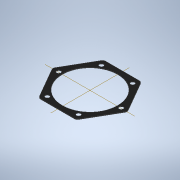
# Autodesk Inventor part: crankcase gasket
Saved by Autodesk Inventor 2021.1 (Build 251245000, 245)
## iProperties
Created: 2020-08-30
Part Number: crankcase gasket
Material: Rubber
Document SubType Name: Sheet Metal
Designer: Vamshi
Mass: 47.7006 g
Surface Area: 454.102 cm^2
Volume: 51.291 cm^3
Density: 0.93 g/cm^3
Sheet Metal Rule: Default
Appearance: Rubber - Black
Author: Vamshi
Autodesk Inventor part; units mm, degrees
ref_plane "YZ Plane" through (0, 0, 0) normal (1, 0, 0) x (0, 1, 0)
ref_plane "XZ Plane" through (0, 0, 0) normal (0, 1, 0) x (-1, 0, 0)
ref_plane "XY Plane" through (0, 0, 0) normal (0, 0, 1) x (1, 0, 0)
sketch "Sketch1" plane through (0, 0, 0) normal (0, 0, 1) x (1, 0, 0)
  line L0 (151.7796, -6.35) -> (81.3891, -128.27)
  line L1 (70.3905, -134.62) -> (-70.3905, -134.62)
  line L2 (-81.3891, -128.27) -> (-151.7796, -6.35)
  line L3 (-151.7796, 6.35) -> (-81.3891, 128.27)
  line L4 (-70.3905, 134.62) -> (70.3905, 134.62)
  line L5 (81.3891, 128.27) -> (151.7796, 6.35)
  arc A0 (-70.3905, 134.62) -> (-81.3891, 128.27) centre (-70.3905, 121.92) ccw
  arc A1 (81.3891, 128.27) -> (70.3905, 134.62) centre (70.3905, 121.92) ccw
  arc A2 (151.7796, -6.35) -> (151.7796, 6.35) centre (140.7811, 0) ccw
  arc A3 (70.3905, -134.62) -> (81.3891, -128.27) centre (70.3905, -121.92) ccw
  arc A4 (-81.3891, -128.27) -> (-70.3905, -134.62) centre (-70.3905, -121.92) ccw
  arc A5 (-151.7796, 6.35) -> (-151.7796, -6.35) centre (-140.7811, 0) ccw
  circle A6 centre (0, 0) radius 129.54 construction
  circle A7 centre (0, 0) radius 114.3
  circle A8 centre (-129.54, 0) radius 8.89
  circle A9 centre (-64.77, -112.1849) radius 8.89
  circle A10 centre (64.77, -112.1849) radius 8.89
  circle A11 centre (129.54, 0) radius 8.89
  circle A12 centre (64.77, 112.1849) radius 8.89
  circle A13 centre (-64.77, 112.1849) radius 8.89
  point P0 (155.4458, 0)
  point P1 (77.7229, -134.62)
  point P2 (-77.7229, -134.62)
  point P3 (-155.4458, 0)
  point P4 (-77.7229, 134.62)
  point P5 (77.7229, 134.62)
  dimension "d2" = 259.08
  dimension "d0" = 269.24
  dimension "d1" = 12.7
  dimension "d3" = 228.6
  dimension "d4" = 17.78
  dimension "d7" = 360
  constraints: 13 centre point, 12 end point, 12 point on circle, 12 point on line, 12 tangent, 5 equal radius, 3 coincident, 1 horizontal, 1 horizontal alignment, 28 other
  measures "d0" distance between parallel lines of L1 L4
  measures "d1" radius of A0
  measures "d3" diameter of A7
  measures "d4" diameter of A8
extrude "Extrusion1" add sketch "Sketch1" along normal blind 2.54
equation "\"BendRadius\" = Thickness"
equation "\"BendReliefWidth\" = Thickness"
equation "\"BendReliefDepth\" = 0.5 * Thickness"
equation "\"CornerReliefSize\" = 4 * Thickness"
equation "\"MinimumRemnant\" = 2 * Thickness"
equation "\"TransitionRadius\" = BendRadius"
equation "\"JacobiRadiusSize\" = BendRadius"
equation "\"GapSize\" = Thickness"
equation "\"Thickness\" = 3.048"
body "Solid1"
